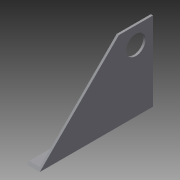
# Autodesk Inventor part: Z-Plate-L
Saved by Autodesk Inventor 2013 (Build 170138000, 138)
## iProperties
Created: 2014-01-24
Part Number: Z-Plate-L
Material: Generic
Document SubType Name: Modeling
Designer: Jarod
Density: 1 g/cm^3
Author: Jarod
Autodesk Inventor part; units mm, degrees
ref_plane "YZ Plane" through (0, 0, 0) normal (1, 0, 0) x (0, 1, 0)
ref_plane "XZ Plane" through (0, 0, 0) normal (0, 1, 0) x (-1, 0, 0)
ref_plane "XY Plane" through (0, 0, 0) normal (0, 0, 1) x (1, 0, 0)
sketch "Sketch1" plane through (0, 0, 0) normal (1, 0, 0) x (0, 1, 0)
  line L0 (0, 0) -> (92.075, 0)
  line L1 (0, 0) -> (92.075, 0) construction
  circle A0 centre (92.075, 0) radius 14.2875
  line L2 (92.075, 0) -> (117.475, 0)
  line L3 (92.075, 0) -> (117.475, 0) construction
  line L4 (117.475, 0) -> (117.475, -25.4)
  line L5 (117.475, -25.4) -> (0, -25.4)
  line L6 (0, -25.4) -> (0, 0)
  line L7 (117.475, 0) -> (117.475, 25.4)
  line L8 (117.475, 0) -> (142.875, 0) construction
  line L9 (117.475, 25.4) -> (0, 142.875)
  line L10 (0, 142.875) -> (0, 0)
  dimension "d0" = 92.075
  dimension "d1" = 0
  dimension "d2" = 28.575
  dimension "d3" = 25.4
  dimension "d4" = 0
  dimension "d5" = 25.4
  dimension "d6" = 90
  dimension "d7" = 25.4
  dimension "d8" = 90
  dimension "d9" = 135
  constraints: 22 end point, 4 horizontal, 3 equal length, 3 parallel, 1 centre point, 1 coincident, 1 collinear, 1 perpendicular
  measures "d0" distance of L0.start L0.end
  measures "d1" distance between parallel lines of L0 L1
  measures "d2" diameter of A0
  measures "d3" distance of L2.start L2.end
  measures "d4" distance between parallel lines of L2 L3
  measures "d5" distance of L3.end L4.end
  measures "d6" angle of L4 L5
  measures "d7" distance of L3.end L7.end
  measures "d8" angle of L8 L7
  measures "d9" angle of L9 L7
extrude "Extrusion1" add sketch "Sketch1" along normal blind 3.175 contours L10 L9 L7 L2 A0 L0 | L0 A0 L2 L4 L5 L6
sketch "Sketch2" plane through (0, 0, 0) normal (-1, 0, 0) x (0, 0, 1)
  line L0 (142.875, 0) -> (-25.4, 0) projected
  line L1 (25.4, 117.475) -> (142.875, 0) projected
  line L2 (-25.4, 0) -> (-25.4, 117.475) projected
  line L3 (-25.4, 0) -> (-25.4, 3.175)
  line L4 (-25.4, 0) -> (-22.225, 0) construction
  line L5 (-25.4, 3.175) -> (139.7, 3.175)
  point P0 (0, 0)
  dimension "d12" = 3.175
  dimension "d13" = 90
  constraints: 6 end point, 2 perpendicular, 1 collinear, 1 horizontal, 1 point on line
  measures "d12" distance of L0.end L3.end
  measures "d13" angle of L4 L3
extrude "Extrusion2" add sketch "Sketch2" along normal blind 15.875
body "Solid1"
